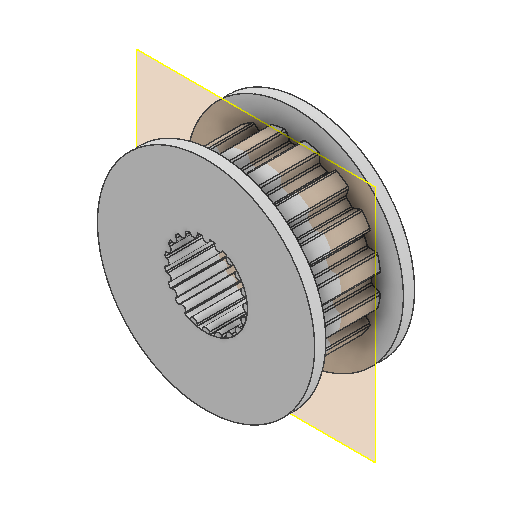
# Autodesk Inventor part: Diff Small Pulley
Saved by Autodesk Inventor 2025.2 (Build 292293000, 293)
## iProperties
Created: 2025-02-20
Part Number: Diff Small Pulley
Material: Generic
Document SubType Name: Modeling
Designer: Jakeg
Density: 1 g/cm^3
Appearance: Default
Author: Jakeg
Autodesk Inventor part; units mm, degrees
ref_plane "YZ Plane" through (0, 0, 0) normal (1, 0, 0) x (0, 1, 0)
ref_plane "XZ Plane" through (0, 0, 0) normal (0, 1, 0) x (-1, 0, 0)
ref_plane "XY Plane" through (0, 0, 0) normal (0, 0, 1) x (1, 0, 0)
sketch "Sketch1" plane through (0, 0, 0) normal (0, 0, 1) x (1, 0, 0)
  circle A0 centre (0, 0) radius 6
  circle A1 centre (0, 0) radius 15.75
  dimension "d0" = 12
  dimension "d1" = 31.5
  constraints: 2 centre point, 2 coincident
  measures "d0" diameter of A0
  measures "d1" diameter of A1
extrude "Extrusion1" add sketch "Sketch1" along normal blind 14.5
ref_plane "Work Plane1" through (0, 0, 7.25) normal (0, 0, 1) x (1, 0, 0)
sketch "Sketch2" plane through (0, 0, 7.25) normal (0, 0, 1) x (1, 0, 0)
  circle A0 centre (0, 0) radius 12.5
  circle A1 centre (0, 0) radius 15.75
  dimension "d5" = 25
  constraints: 2 centre point, 2 coincident
  measures "d5" diameter of A0
extrude "Extrusion2" cut sketch "Sketch2" along normal mid plane 11.25
sketch "Sketch3" plane through (0, 0, 14.5) normal (0, 0, 1) x (1, 0, 0)
  arc A0 (-1.277994, -5.546817) -> (-2.226914, -5.238494) centre (-1.827608, -5.623954) ccw
  arc A1 (-1.278569, -5.828822) -> (-1.277994, -5.546817) centre (-2.268289, -5.685804) ccw
  arc A2 (-1.278569, -5.828822) -> (-1.158554, -5.997554) centre (-1.130111, -5.850275) ccw
  arc A3 (-1.158554, -5.997554) -> (-0.751747, -6.061994) centre (0, 0) ccw
  arc A4 (-0.751747, -6.061994) -> (-0.585466, -5.938608) centre (-0.733287, -5.913134) ccw
  arc A5 (-0.498868, -5.670227) -> (-0.585466, -5.938608) centre (0.400009, -6.108429) ccw
  arc A6 (0.498885, -5.670227) -> (-0.498868, -5.670227) centre (0.000009, -5.913429) ccw
  arc A7 (0.585484, -5.938608) -> (0.498885, -5.670227) centre (-0.399991, -6.108429) ccw
  arc A8 (0.585484, -5.938608) -> (0.751765, -6.061994) centre (0.733305, -5.913134) ccw
  arc A9 (0.751765, -6.061994) -> (1.158327, -5.997601) centre (0.000009, 0.000071) ccw
  arc A10 (1.158327, -5.997601) -> (1.278342, -5.82887) centre (1.129884, -5.850323) ccw
  arc A11 (1.277768, -5.546864) -> (1.278342, -5.82887) centre (2.268062, -5.685851) ccw
  arc A12 (2.226687, -5.238541) -> (1.277768, -5.546864) centre (1.827381, -5.624002) ccw
  arc A13 (2.391981, -5.467026) -> (2.226687, -5.238541) centre (1.507217, -5.933065) ccw
  arc A14 (2.391981, -5.467026) -> (2.588253, -5.53299) centre (2.524696, -5.397121) ccw
  arc A15 (2.588253, -5.53299) -> (2.955018, -5.346114) centre (0.000009, 0.000071) ccw
  arc A16 (2.955018, -5.346114) -> (3.017017, -5.148554) centre (2.882455, -5.214833) ccw
  arc A17 (2.929327, -4.880528) -> (3.017017, -5.148554) centre (3.914102, -4.706695) ccw
  arc A18 (3.736526, -4.294064) -> (2.929327, -4.880528) centre (3.475877, -4.784051) ccw
  arc A19 (3.964336, -4.460287) -> (3.736526, -4.294064) centre (3.266888, -5.176923) ccw
  arc A20 (3.964336, -4.460287) -> (4.171385, -4.462372) centre (4.068953, -4.352792) ccw
  arc A21 (4.171385, -4.462372) -> (4.462451, -4.171305) centre (0.000009, 0.000071) ccw
  arc A22 (4.462451, -4.171305) -> (4.460367, -3.964256) centre (4.352872, -4.068873) ccw
  arc A23 (4.294144, -3.736446) -> (4.460367, -3.964256) centre (5.177003, -3.266808) ccw
  arc A24 (4.880608, -2.929247) -> (4.294144, -3.736446) centre (4.784131, -3.475797) ccw
  arc A25 (5.148634, -3.016938) -> (4.880608, -2.929247) centre (4.706775, -3.914022) ccw
  arc A26 (5.148634, -3.016938) -> (5.346194, -2.954938) centre (5.214913, -2.882375) ccw
  arc A27 (5.346194, -2.954938) -> (5.53307, -2.588173) centre (0.000009, 0.000071) ccw
  arc A28 (5.53307, -2.588173) -> (5.467106, -2.391901) centre (5.3972, -2.524616) ccw
  arc A29 (5.238621, -2.226607) -> (5.467106, -2.391901) centre (5.933144, -1.507137) ccw
  arc A30 (5.546944, -1.277688) -> (5.238621, -2.226607) centre (5.624082, -1.827301) ccw
  arc A31 (5.82895, -1.278262) -> (5.546944, -1.277688) centre (5.685931, -2.267982) ccw
  arc A32 (5.82895, -1.278262) -> (5.997681, -1.158248) centre (5.850402, -1.129804) ccw
  arc A33 (5.997681, -1.158248) -> (6.062074, -0.751685) centre (0.000009, 0.000071) ccw
  arc A34 (6.062074, -0.751685) -> (5.938687, -0.585404) centre (5.913214, -0.733225) ccw
  arc A35 (5.663912, -0.495883) -> (5.938687, -0.585404) centre (6.107819, 0.40019) ccw
  arc A36 (5.663912, 0.50187) -> (5.663912, -0.495883) centre (5.907114, 0.002993) ccw
  arc A37 (5.932293, 0.588468) -> (5.663912, 0.50187) centre (6.102114, -0.397007) ccw
  arc A38 (5.932293, 0.588468) -> (6.05568, 0.754749) centre (5.90682, 0.736289) ccw
  arc A39 (6.05568, 0.754749) -> (5.991286, 1.161312) centre (-0.006386, 0.002993) ccw
  arc A40 (5.991286, 1.161312) -> (5.822555, 1.281326) centre (5.844008, 1.132868) ccw
  arc A41 (5.540549, 1.280752) -> (5.822555, 1.281326) centre (5.679536, 2.271046) ccw
  arc A42 (5.232227, 2.229671) -> (5.540549, 1.280752) centre (5.617687, 1.830365) ccw
  arc A43 (5.460712, 2.394966) -> (5.232227, 2.229671) centre (5.92675, 1.510201) ccw
  arc A44 (5.460712, 2.394966) -> (5.526676, 2.591237) centre (5.390806, 2.52768) ccw
  arc A45 (5.526676, 2.591237) -> (5.339799, 2.958002) centre (-0.006386, 0.002993) ccw
  arc A46 (5.339799, 2.958002) -> (5.14224, 3.020002) centre (5.208519, 2.885439) ccw
  arc A47 (4.874214, 2.932311) -> (5.14224, 3.020002) centre (4.700381, 3.917086) ccw
  arc A48 (4.287749, 3.73951) -> (4.874214, 2.932311) centre (4.777736, 3.478861) ccw
  arc A49 (4.453973, 3.96732) -> (4.287749, 3.73951) centre (5.170609, 3.269873) ccw
  arc A50 (4.453973, 3.96732) -> (4.456057, 4.174369) centre (4.346477, 4.071937) ccw
  arc A51 (4.456057, 4.174369) -> (4.16499, 4.465436) centre (-0.006386, 0.002993) ccw
  arc A52 (4.16499, 4.465436) -> (3.957941, 4.463352) centre (4.062558, 4.355856) ccw
  arc A53 (3.730131, 4.297128) -> (3.957941, 4.463352) centre (3.260494, 5.179988) ccw
  arc A54 (2.922932, 4.883593) -> (3.730131, 4.297128) centre (3.469482, 4.787115) ccw
  arc A55 (3.010623, 5.151619) -> (2.922932, 4.883593) centre (3.907707, 4.709759) ccw
  arc A56 (3.010623, 5.151619) -> (2.948623, 5.349178) centre (2.87606, 5.217898) ccw
  arc A57 (2.948623, 5.349178) -> (2.581858, 5.536054) centre (-0.006386, 0.002993) ccw
  arc A58 (2.581858, 5.536054) -> (2.385587, 5.470091) centre (2.518301, 5.400185) ccw
  arc A59 (2.220292, 5.241606) -> (2.385587, 5.470091) centre (1.500822, 5.936129) ccw
  arc A60 (1.271373, 5.549928) -> (2.220292, 5.241606) centre (1.820986, 5.627066) ccw
  arc A61 (1.271947, 5.831934) -> (1.271373, 5.549928) centre (2.261667, 5.688915) ccw
  arc A62 (1.271947, 5.831934) -> (1.151933, 6.000665) centre (1.123489, 5.853387) ccw
  arc A63 (1.151933, 6.000665) -> (0.745371, 6.065058) centre (-0.006386, 0.002993) ccw
  arc A64 (0.745371, 6.065058) -> (0.579089, 5.941672) centre (0.72691, 5.916199) ccw
  arc A65 (0.492491, 5.673291) -> (0.579089, 5.941672) centre (-0.406386, 6.111493) ccw
  arc A66 (-0.505262, 5.673291) -> (0.492491, 5.673291) centre (-0.006386, 5.916493) ccw
  arc A67 (-0.591861, 5.941672) -> (-0.505262, 5.673291) centre (0.393614, 6.111493) ccw
  arc A68 (-0.591861, 5.941672) -> (-0.758142, 6.065058) centre (-0.739682, 5.916199) ccw
  arc A69 (-0.758142, 6.065058) -> (-1.164704, 6.000665) centre (-0.006386, 0.002993) ccw
  arc A70 (-1.164704, 6.000665) -> (-1.284719, 5.831934) centre (-1.136261, 5.853387) ccw
  arc A71 (-1.284144, 5.549928) -> (-1.284719, 5.831934) centre (-2.274439, 5.688915) ccw
  arc A72 (-2.233064, 5.241606) -> (-1.284144, 5.549928) centre (-1.833758, 5.627066) ccw
  arc A73 (-2.398358, 5.470091) -> (-2.233064, 5.241606) centre (-1.513593, 5.936129) ccw
  arc A74 (-2.398358, 5.470091) -> (-2.594629, 5.536054) centre (-2.531073, 5.400185) ccw
  arc A75 (-2.594629, 5.536054) -> (-2.961395, 5.349178) centre (-0.006386, 0.002993) ccw
  arc A76 (-2.961395, 5.349178) -> (-3.023394, 5.151619) centre (-2.888832, 5.217898) ccw
  arc A77 (-2.935704, 4.883593) -> (-3.023394, 5.151619) centre (-3.920479, 4.709759) ccw
  arc A78 (-3.742903, 4.297128) -> (-2.935704, 4.883593) centre (-3.482254, 4.787115) ccw
  arc A79 (-3.970713, 4.463352) -> (-3.742903, 4.297128) centre (-3.273265, 5.179988) ccw
  arc A80 (-3.970713, 4.463352) -> (-4.177762, 4.465436) centre (-4.07533, 4.355856) ccw
  arc A81 (-4.177762, 4.465436) -> (-4.468828, 4.174369) centre (-0.006386, 0.002993) ccw
  arc A82 (-4.468828, 4.174369) -> (-4.466744, 3.96732) centre (-4.359249, 4.071937) ccw
  arc A83 (-4.300521, 3.73951) -> (-4.466744, 3.96732) centre (-5.18338, 3.269873) ccw
  arc A84 (-4.886985, 2.932311) -> (-4.300521, 3.73951) centre (-4.790508, 3.478861) ccw
  arc A85 (-5.155011, 3.020002) -> (-4.886985, 2.932311) centre (-4.713152, 3.917086) ccw
  arc A86 (-5.155011, 3.020002) -> (-5.352571, 2.958002) centre (-5.22129, 2.885439) ccw
  arc A87 (-5.352571, 2.958002) -> (-5.539447, 2.591237) centre (-0.006386, 0.002993) ccw
  arc A88 (-5.539447, 2.591237) -> (-5.473483, 2.394966) centre (-5.403577, 2.52768) ccw
  arc A89 (-5.244998, 2.229671) -> (-5.473483, 2.394966) centre (-5.939521, 1.510201) ccw
  arc A90 (-5.553321, 1.280752) -> (-5.244998, 2.229671) centre (-5.630458, 1.830365) ccw
  arc A91 (-5.835326, 1.281326) -> (-5.553321, 1.280752) centre (-5.692308, 2.271046) ccw
  arc A92 (-5.835326, 1.281326) -> (-6.004058, 1.161312) centre (-5.856779, 1.132868) ccw
  arc A93 (-6.004058, 1.161312) -> (-6.068451, 0.754749) centre (-0.006386, 0.002993) ccw
  arc A94 (-6.068451, 0.754749) -> (-5.945064, 0.588468) centre (-5.919591, 0.736289) ccw
  arc A95 (-5.676683, 0.50187) -> (-5.945064, 0.588468) centre (-6.114886, -0.397007) ccw
  arc A96 (-5.676683, -0.495883) -> (-5.676683, 0.50187) centre (-5.919886, 0.002993) ccw
  arc A97 (-5.945064, -0.582482) -> (-5.676683, -0.495883) centre (-6.114886, 0.402993) ccw
  arc A98 (-5.945064, -0.582482) -> (-6.068451, -0.748763) centre (-5.919591, -0.730303) ccw
  arc A99 (-6.068451, -0.748763) -> (-6.004058, -1.155325) centre (-0.006386, 0.002993) ccw
  arc A100 (-6.004058, -1.155325) -> (-5.835326, -1.27534) centre (-5.856779, -1.126882) ccw
  arc A101 (-5.553321, -1.274765) -> (-5.835326, -1.27534) centre (-5.692308, -2.26506) ccw
  arc A102 (-5.244998, -2.223685) -> (-5.553321, -1.274765) centre (-5.630458, -1.824379) ccw
  arc A103 (-5.473483, -2.388979) -> (-5.244998, -2.223685) centre (-5.939521, -1.504214) ccw
  arc A104 (-5.473483, -2.388979) -> (-5.539447, -2.585251) centre (-5.403577, -2.521694) ccw
  arc A105 (-5.539447, -2.585251) -> (-5.352571, -2.952016) centre (-0.006386, 0.002993) ccw
  arc A106 (-5.352571, -2.952016) -> (-5.155011, -3.014015) centre (-5.22129, -2.879453) ccw
  arc A107 (-4.886985, -2.926325) -> (-5.155011, -3.014015) centre (-4.713152, -3.9111) ccw
  arc A108 (-4.300521, -3.733524) -> (-4.886985, -2.926325) centre (-4.790508, -3.472875) ccw
  arc A109 (-4.466744, -3.961334) -> (-4.300521, -3.733524) centre (-5.18338, -3.263886) ccw
  arc A110 (-4.466744, -3.961334) -> (-4.468828, -4.168383) centre (-4.359249, -4.065951) ccw
  arc A111 (-4.468828, -4.168383) -> (-4.177762, -4.459449) centre (-0.006386, 0.002993) ccw
  arc A112 (-4.177762, -4.459449) -> (-3.970713, -4.457365) centre (-4.07533, -4.34987) ccw
  arc A113 (-3.742903, -4.291142) -> (-3.970713, -4.457365) centre (-3.273265, -5.174001) ccw
  arc A114 (-2.935704, -4.877606) -> (-3.742903, -4.291142) centre (-3.482254, -4.781129) ccw
  arc A115 (-3.023394, -5.145632) -> (-2.935704, -4.877606) centre (-3.920479, -4.703773) ccw
  arc A116 (-3.023394, -5.145632) -> (-2.961395, -5.343192) centre (-2.888832, -5.211911) ccw
  arc A117 (-2.961395, -5.343192) -> (-2.58848, -5.532943) centre (-0.005971, 0.003744) ccw
  arc A118 (-2.58848, -5.532943) -> (-2.392208, -5.466979) centre (-2.524923, -5.397073) ccw
  arc A119 (-2.226914, -5.238494) -> (-2.392208, -5.466979) centre (-1.507443, -5.933017) ccw
  circle A120 centre (-0.005971, 0.003744) radius 6
  circle A121 centre (-0.005971, 0.003744) radius 12.520387
  arc A122 (-9.716442, 7.90734) -> (-9.702841, 7.703356) centre (-9.600106, 7.812651) ccw
  arc A123 (-9.536618, 7.475546) -> (-9.702841, 7.703356) centre (-10.419477, 7.005908) ccw
  arc A124 (-10.123082, 6.668347) -> (-9.536618, 7.475546) centre (-10.026605, 7.214897) ccw
  arc A125 (-10.391108, 6.756038) -> (-10.123082, 6.668347) centre (-9.949249, 7.653122) ccw
  arc A126 (-10.391108, 6.756038) -> (-10.584118, 6.70172) centre (-10.457387, 6.621475) ccw
  arc A127 (-11.383003, 4.903875) -> (-11.564057, 4.817719) centre (-11.425588, 4.760046) ccw
  arc A128 (-11.383003, 4.903875) -> (-11.104013, 4.862742) centre (-11.099108, 5.86273) ccw
  arc A129 (-11.104013, 4.862742) -> (-10.662401, 5.757443) centre (-11.10129, 5.417735) ccw
  arc A130 (-10.912613, 6.152636) -> (-10.864734, 5.953884) centre (-10.781948, 6.07897) ccw
  arc A131 (-10.662401, 5.757443) -> (-10.864734, 5.953884) centre (-11.453193, 5.145357) ccw
  arc A132 (-12.047614, 2.910722) -> (-12.211503, 2.795208) centre (-12.065279, 2.761766) ccw
  arc A133 (-12.047614, 2.910722) -> (-11.765685, 2.917331) centre (-11.929849, 3.903764) ccw
  arc A134 (-11.765685, 2.917331) -> (-11.481631, 3.873795) centre (-11.856796, 3.464801) ccw
  arc A135 (-11.795031, 4.221017) -> (-11.714252, 4.033216) centre (-11.653796, 4.170494) ccw
  arc A136 (-11.481631, 3.873795) -> (-11.714252, 4.033216) centre (-12.157604, 3.136869) ccw
  arc A137 (-12.36582, 0.83392) -> (-12.50783, 0.692369) centre (-12.358057, 0.684121) ccw
  arc A138 (-12.36582, 0.83392) -> (-12.089064, 0.888079) centre (-12.417575, 1.83258) ccw
  arc A139 (-12.089064, 0.888079) -> (-11.970739, 1.878791) centre (-12.271387, 1.412277) ccw
  arc A140 (-12.338312, 2.168054) -> (-12.226956, 1.996606) centre (-12.19057, 2.142126) ccw
  arc A141 (-11.970739, 1.878791) -> (-12.226956, 1.996606) centre (-12.512448, 1.038225) ccw
  arc A142 (-12.328468, -1.266787) -> (-12.444514, -1.430301) centre (-12.295501, -1.413119) ccw
  arc A143 (-12.328468, -1.266787) -> (-12.064846, -1.166634) centre (-12.548252, -0.291239) ccw
  arc A144 (-12.064846, -1.166634) -> (-12.115654, -0.170176) centre (-12.333136, -0.68079) ccw
  arc A145 (-12.526825, 0.052806) -> (-12.388096, -0.097357) centre (-12.376826, 0.05222) ccw
  arc A146 (-12.115654, -0.170176) -> (-12.388096, -0.097357) centre (-12.507514, -1.090201) ccw
  arc A147 (-11.936633, -3.330965) -> (-12.023374, -3.511738) centre (-11.879409, -3.46962) ccw
  arc A148 (-11.936633, -3.330965) -> (-11.693728, -3.1877) centre (-12.318124, -2.406592) ccw
  arc A149 (-11.693728, -3.1877) -> (-11.912207, -2.214161) centre (-12.040267, -2.754185) ccw
  arc A150 (-12.355149, -2.063875) -> (-12.193038, -2.188432) centre (-12.207208, -2.039103) ccw
  arc A151 (-11.912207, -2.214161) -> (-12.193038, -2.188432) centre (-12.142946, -3.187177) ccw
  arc A152 (-11.201585, -5.29923) -> (-11.256529, -5.492063) centre (-11.121752, -5.426221) ccw
  arc A153 (-11.201585, -5.29923) -> (-10.986386, -5.116975) centre (-11.733809, -4.452626) ccw
  arc A154 (-10.986386, -5.116975) -> (-11.366252, -4.194363) centre (-11.401206, -4.748261) ccw
  arc A155 (-11.82822, -4.121096) -> (-11.647391, -4.216465) centre (-11.686594, -4.071678) ccw
  arc A156 (-11.366252, -4.194363) -> (-11.647391, -4.216465) centre (-11.429232, -5.192378) ccw
  arc A157 (-10.144472, -7.11496) -> (-10.166036, -7.314305) centre (-10.044326, -7.226632) ccw
  arc A158 (-10.144472, -7.11496) -> (-9.96317, -6.898958) centre (-10.812117, -6.37048) ccw
  arc A159 (-9.96317, -6.898958) -> (-10.493494, -6.053815) centre (-10.434336, -6.605653) ccw
  arc A160 (-10.9612, -6.059674) -> (-10.766854, -6.123111) centre (-10.829962, -5.987033) ccw
  arc A161 (-10.493494, -6.053815) -> (-10.766854, -6.123111) centre (-10.386902, -7.048118) ccw
  arc A162 (-8.795705, -8.72592) -> (-8.78327, -8.926042) centre (-8.678126, -8.819061) ccw
  arc A163 (-8.795705, -8.72592) -> (-8.653515, -8.482384) centre (-9.579564, -8.104981) ccw
  arc A164 (-8.653515, -8.482384) -> (-9.319041, -7.739023) centre (-9.167472, -8.272926) ccw
  arc A165 (-9.779029, -7.823841) -> (-9.576758, -7.853521) centre (-9.661956, -7.730065) ccw
  arc A166 (-9.319041, -7.739023) -> (-9.576758, -7.853521) centre (-9.045944, -8.70101) ccw
  arc A167 (-7.194085, -10.085765) -> (-7.148008, -10.280906) centre (-7.062457, -10.157695) ccw
  arc A168 (-7.194085, -10.085765) -> (-7.095098, -9.821702) centre (-8.071608, -9.60623) ccw
  arc A169 (-7.095098, -9.821702) -> (-7.87668, -9.201508) centre (-7.637061, -9.702115) ccw
  arc A170 (-8.315717, -9.362844) -> (-8.111339, -9.357913) centre (-8.216176, -9.250631) ccw
  arc A171 (-7.87668, -9.201508) -> (-8.111339, -9.357913) centre (-7.444935, -10.103503) ccw
  arc A172 (-5.385688, -11.155374) -> (-5.307295, -11.339922) centre (-5.243797, -11.204025) ccw
  arc A173 (-5.385688, -11.155374) -> (-5.332752, -10.878381) centre (-6.331631, -10.83104) ccw
  arc A174 (-5.332752, -10.878381) -> (-6.207905, -10.399195) centre (-5.88713, -10.852107) ccw
  arc A175 (-6.61336, -10.632409) -> (-6.412756, -10.593008) centre (-6.534215, -10.504988) ccw
  arc A176 (-6.207905, -10.399195) -> (-6.412756, -10.593008) centre (-5.629932, -11.215252) ccw
  arc A177 (-3.422539, -11.903978) -> (-3.314084, -12.072622) centre (-3.274466, -11.927949) ccw
  arc A178 (-3.422539, -11.903978) -> (-3.417176, -11.622023) centre (-4.409688, -11.744174) ccw
  arc A179 (-3.417176, -11.622023) -> (-4.360723, -11.297631) centre (-3.96802, -11.689816) ccw
  arc A180 (-4.720933, -11.596012) -> (-4.529873, -11.523276) centre (-4.664461, -11.457049) ccw
  arc A181 (-4.360723, -11.297631) -> (-4.529873, -11.523276) centre (-3.65315, -12.004271) ccw
  arc A182 (-1.361113, -12.31004) -> (-1.225717, -12.457929) centre (-1.211119, -12.308641) ccw
  arc A183 (-1.361113, -12.31004) -> (-1.403478, -12.031234) centre (-2.361069, -12.319363) ccw
  arc A184 (-1.403478, -12.031234) -> (-2.388275, -11.870968) centre (-1.934941, -12.191145) ccw
  arc A185 (-2.692878, -12.225933) -> (-2.516858, -12.121955) centre (-2.660702, -12.079425) ccw
  arc A186 (-2.388275, -11.870968) -> (-2.516858, -12.121955) centre (-1.571457, -12.447864) ccw
  arc A187 (0.739287, -12.361878) -> (0.897728, -12.484758) centre (0.886886, -12.335151) ccw
  arc A188 (0.739287, -12.361878) -> (0.650412, -12.094242) centre (-0.244711, -12.54006) ccw
  arc A189 (0.650412, -12.094242) -> (-0.347304, -12.102714) centre (0.153619, -12.341671) ccw
  arc A190 (-0.587536, -12.504051) -> (-0.431621, -12.37182) centre (-0.580584, -12.354212) ccw
  arc A191 (-0.347304, -12.102714) -> (-0.431621, -12.37182) centre (0.55526, -12.533268) ccw
  arc A192 (2.818234, -12.058001) -> (2.995163, -12.152337) centre (2.959194, -12.006714) ccw
  arc A193 (2.818234, -12.058001) -> (2.685408, -11.809235) centre (1.878504, -12.399917) ccw
  arc A194 (2.685408, -11.809235) -> (1.703474, -11.9862) centre (2.237576, -12.137064) ccw
  arc A195 (1.534524, -12.422363) -> (1.665849, -12.265685) centre (1.516053, -12.273505) ccw
  arc A196 (1.703474, -11.9862) -> (1.665849, -12.265685) centre (2.66582, -12.258027) ccw
  arc A197 (4.815922, -11.407152) -> (5.00625, -11.47023) centre (4.946187, -11.33278) ccw
  arc A198 (4.815922, -11.407152) -> (4.642965, -11.184411) centre (3.947493, -11.902965) ccw
  arc A199 (4.642965, -11.184411) -> (3.705062, -11.524778) centre (4.256978, -11.583209) ccw
  arc A200 (3.612255, -11.983221) -> (3.715212, -11.806602) centre (3.568893, -11.839625) ccw
  arc A201 (3.705062, -11.524778) -> (3.715212, -11.806602) centre (4.699505, -11.630058) ccw
  arc A202 (6.674882, -10.428053) -> (6.873132, -10.458058) centre (6.790704, -10.332736) ccw
  arc A203 (6.674882, -10.428053) -> (6.466769, -10.237747) centre (5.902737, -11.0635) ccw
  arc A204 (6.466769, -10.237747) -> (5.599879, -10.731724) centre (6.153731, -10.69604) ccw
  arc A205 (5.585884, -11.199257) -> (5.657512, -11.007779) centre (5.518878, -11.065055) ccw
  arc A206 (5.599879, -10.731724) -> (5.657512, -11.007779) centre (6.59781, -10.667428) ccw
  arc A207 (8.341633, -9.148872) -> (8.542102, -9.144942) centre (8.43968, -9.035353) ccw
  arc A208 (8.341633, -9.148872) -> (8.104352, -8.996475) centre (7.687986, -9.905672) ccw
  arc A209 (8.104352, -8.996475) -> (7.333414, -9.629851) centre (7.873269, -9.501079) ccw
  arc A210 (7.398634, -10.093025) -> (7.436871, -9.892195) centre (7.309911, -9.972077) ccw
  arc A211 (7.333414, -9.629851) -> (7.436871, -9.892195) centre (8.306125, -9.397829) ccw
  arc A212 (9.768227, -7.606409) -> (9.965149, -7.568655) centre (9.845679, -7.477952) ccw
  arc A213 (9.768227, -7.606409) -> (9.508604, -7.496304) centre (9.251882, -8.462789) ccw
  arc A214 (9.508604, -7.496304) -> (8.855797, -8.25086) centre (9.366123, -8.032703) ccw
  arc A215 (8.998355, -8.696348) -> (9.002102, -8.491946) centre (8.890468, -8.592135) ccw
  arc A216 (8.855797, -8.25086) -> (9.002102, -8.491946) centre (9.775304, -7.857786) ccw
  arc A217 (10.913624, -5.845037) -> (11.101332, -5.774547) centre (10.968252, -5.705338) ccw
  arc A218 (10.913624, -5.845037) -> (10.639127, -5.780393) centre (10.549434, -6.776362) ccw
  arc A219 (10.639127, -5.780393) -> (10.12323, -6.634419) centre (10.589347, -6.333156) ccw
  arc A220 (10.339025, -7.049408) -> (10.308175, -6.847312) centre (10.215078, -6.964926) ccw
  arc A221 (10.12323, -6.634419) -> (10.308175, -6.847312) centre (10.963081, -6.091602) ccw
  arc A222 (11.744871, -3.915428) -> (11.917967, -3.814229) centre (11.775105, -3.768506) ccw
  arc A223 (11.744871, -3.915428) -> (11.463398, -3.898104) centre (11.543315, -4.894905) ccw
  arc A224 (11.463398, -3.898104) -> (11.099253, -4.827033) centre (11.507752, -4.451328) ccw
  arc A225 (11.382078, -5.199582) -> (11.317516, -5.005607) centre (11.245636, -5.137263) ccw
  arc A226 (11.099253, -4.827033) -> (11.317516, -5.005607) centre (11.835287, -4.150088) ccw
  arc A227 (12.238057, -1.873093) -> (12.391559, -1.744096) centre (12.243025, -1.723175) ccw
  arc A228 (12.238057, -1.873093) -> (11.957704, -1.903587) centre (12.204932, -2.872544) ccw
  arc A229 (11.957704, -1.903587) -> (11.755787, -2.880695) centre (12.094915, -2.441358) ccw
  arc A230 (12.097504, -3.200088) -> (12.00109, -3.019814) centre (11.952493, -3.161724) ccw
  arc A231 (11.755787, -2.880695) -> (12.00109, -3.019814) centre (12.366829, -2.089097) ccw
  arc A232 (12.378992, 0.223214) -> (12.508486, 0.376297) centre (12.358553, 0.371815) ccw
  arc A233 (12.378992, 0.223214) -> (12.107825, 0.145778) centre (12.515252, -0.76746) ccw
  arc A234 (12.107825, 0.145778) -> (12.073945, -0.851399) centre (12.333947, -0.361069) ccw
  arc A235 (12.464724, -1.108448) -> (12.33923, -0.947061) centre (12.315316, -1.095142) ccw
  arc A236 (12.073945, -0.851399) -> (12.33923, -0.947061) centre (12.542417, 0.032079) ccw
  arc A237 (12.163622, 2.313185) -> (12.265382, 2.485951) centre (12.118363, 2.456194) ccw
  arc A238 (12.163622, 2.313185) -> (11.909442, 2.191036) centre (12.465346, 1.35979) ccw
  arc A239 (11.909442, 2.191036) -> (12.044573, 1.202476) centre (12.217969, 1.729694) ccw
  arc A240 (12.473173, 1.015167) -> (12.32221, 1.153024) centre (12.323665, 1.003031) ccw
  arc A241 (12.044573, 1.202476) -> (12.32221, 1.153024) centre (12.356998, 2.152419) ccw
  arc A242 (11.598143, 4.336696) -> (11.669242, 4.524175) centre (11.529367, 4.469999) ccw
  arc A243 (11.598143, 4.336696) -> (11.368263, 4.173348) centre (12.056652, 3.448006) ccw
  arc A244 (11.368263, 4.173348) -> (11.668517, 3.221845) centre (11.750319, 3.770783) ccw
  arc A245 (12.122608, 3.109664) -> (11.950518, 3.220025) centre (11.977301, 3.072435) ccw
  arc A246 (11.668517, 3.221845) -> (11.950518, 3.220025) centre (11.815908, 4.210923) ccw
  arc A247 (10.698823, 6.235535) -> (10.737215, 6.432332) centre (10.608508, 6.355297) ccw
  arc A248 (10.698823, 6.235535) -> (10.499856, 6.035686) centre (11.300926, 5.437116) ccw
  arc A249 (10.499856, 6.035686) -> (10.956596, 5.148613) centre (10.94445, 5.70348) ccw
  arc A250 (11.423114, 5.114787) -> (11.234848, 5.194477) centre (11.286189, 5.053537) ccw
  arc A251 (10.956596, 5.148613) -> (11.234848, 5.194477) centre (10.934711, 6.148373) ccw
  arc A252 (9.491534, 7.955074) -> (9.496115, 8.155529) centre (9.382278, 8.057851) ccw
  arc A253 (9.491534, 7.955074) -> (9.329203, 7.724474) centre (10.21991, 7.269896) ccw
  arc A254 (9.329203, 7.724474) -> (9.92929, 6.92735) centre (9.823545, 7.472184) ccw
  arc A255 (10.394813, 6.972853) -> (10.195788, 7.01958) centre (10.270209, 6.889344) ccw
  arc A256 (9.92929, 6.92735) -> (10.195788, 7.01958) centre (9.738759, 7.909032) ccw
  arc A257 (8.011007, 9.445847) -> (7.981645, 9.644193) centre (7.885953, 9.528681) ccw
  arc A258 (8.011007, 9.445847) -> (7.889982, 9.19113) centre (8.844701, 8.893621) ccw
  arc A259 (7.889982, 9.19113) -> (8.616152, 8.506887) centre (8.419851, 9.026012) ccw
  arc A260 (9.06729, 8.630409) -> (8.86323, 8.642828) centre (8.958591, 8.527043) ccw
  arc A261 (8.616152, 8.506887) -> (8.86323, 8.642828) centre (8.262457, 9.442248) ccw
  arc A262 (6.299834, 10.664966) -> (6.237373, 10.855497) centre (6.162579, 10.725474) ccw
  arc A263 (6.299834, 10.664966) -> (6.223598, 10.39346) centre (7.214863, 10.261578) ccw
  arc A264 (6.223598, 10.39346) -> (7.054959, 9.841782) centre (6.77375, 10.320265) ccw
  arc A265 (7.478733, 10.03977) -> (7.275509, 10.017524) centre (7.389067, 9.919521) ccw
  arc A266 (7.054959, 9.841782) -> (7.275509, 10.017524) centre (6.548276, 10.703914) ccw
  arc A267 (4.407243, 11.577359) -> (4.313481, 11.754594) centre (4.261736, 11.613801) ccw
  arc A268 (4.407243, 11.577359) -> (4.377988, 11.296875) centre (5.377283, 11.334415) ccw
  arc A269 (4.377988, 11.296875) -> (5.290625, 10.893633) centre (4.932596, 11.317709) ccw
  arc A270 (5.674842, 11.160392) -> (5.478302, 11.104121) centre (5.606789, 11.026718) ccw
  arc A271 (5.290625, 10.893633) -> (5.478302, 11.104121) centre (4.645528, 11.657734) ccw
  arc A272 (2.387679, 12.15678) -> (2.265313, 12.315619) centre (2.238107, 12.168106) ccw
  arc A273 (2.387679, 12.15678) -> (2.406247, 11.875385) centre (3.384824, 12.081267) ccw
  arc A274 (2.406247, 11.875385) -> (3.373905, 11.632181) centre (2.949357, 11.989649) ccw
  arc A275 (3.707514, 11.960035) -> (3.52331, 11.871358) centre (3.66303, 11.816783) ccw
  arc A276 (3.373905, 11.632181) -> (3.52331, 11.871358) centre (2.608954, 12.276269) ccw
  arc A277 (0.299243, 12.386557) -> (0.151793, 12.522432) centre (0.149908, 12.372443) ccw
  arc A278 (0.299243, 12.386557) -> (0.3651, 12.112348) centre (1.294806, 12.480649) ccw
  arc A279 (0.3651, 12.112348) -> (1.359941, 12.036177) centre (0.881087, 12.316755) ccw
  arc A280 (1.633343, 12.415696) -> (1.466775, 12.297164) centre (1.613708, 12.266986) ccw
  arc A281 (1.359941, 12.036177) -> (1.466775, 12.297164) centre (0.497141, 12.541723) ccw
  arc A282 (-1.797986, 12.260082) -> (-1.966278, 12.369083) centre (-1.942787, 12.220934) ccw
  arc A283 (-1.797986, 12.260082) -> (-1.686735, 12.000948) centre (-0.832644, 12.521072) ccw
  arc A284 (-1.686735, 12.000948) -> (-0.693331, 12.094001) centre (-1.212715, 12.289617) ccw
  arc A285 (-0.488, 12.514266) -> (-0.63214, 12.369289) centre (-0.48222, 12.364377) ccw
  arc A286 (-0.693331, 12.094001) -> (-0.63214, 12.369289) centre (-1.629157, 12.446462) ccw
  arc A287 (-3.843673, 11.780993) -> (-4.027966, 11.859985) centre (-3.979776, 11.717937) ccw
  arc A288 (-3.843673, 11.780993) -> (-3.690229, 11.544388) centre (-2.936325, 12.201372) ccw
  arc A289 (-3.690229, 11.544388) -> (-2.72684, 11.803989) centre (-3.271812, 11.909014) ccw
  arc A290 (-2.595488, 12.252909) -> (-2.713053, 12.085658) centre (-2.56446, 12.106153) ccw
  arc A291 (-2.72684, 11.803989) -> (-2.713053, 12.085658) centre (-3.708772, 11.993224) ccw
  arc A292 (-5.778969, 10.963073) -> (-5.97396, 11.009783) centre (-5.902457, 10.877922) ccw
  arc A293 (-5.778969, 10.963073) -> (-5.587745, 10.755803) centre (-4.955716, 11.530748) ccw
  arc A294 (-5.587745, 10.755803) -> (-4.682087, 11.174483) centre (-5.236969, 11.185897) ccw
  arc A295 (-4.628492, 11.639145) -> (-4.7161, 11.454431) centre (-4.573108, 11.499744) ccw
  arc A296 (-4.682087, 11.174483) -> (-4.7161, 11.454431) centre (-5.681875, 11.195049) ccw
  arc A297 (-7.548198, 9.829851) -> (-7.748279, 9.842935) centre (-7.655519, 9.725055) ccw
  arc A298 (-7.548198, 9.829851) -> (-7.324696, 9.657879) centre (-6.832725, 10.52849) ccw
  arc A299 (-7.324696, 9.657879) -> (-6.502822, 10.223594) centre (-7.051652, 10.141068) ccw
  arc A300 (-6.528526, 10.69063) -> (-6.583658, 10.493767) centre (-6.45038, 10.562594) ccw
  arc A301 (-6.502822, 10.223594) -> (-6.583658, 10.493767) centre (-7.491705, 10.074899) ccw
  arc A302 (-9.100463, 8.413928) -> (-9.299877, 8.39301) centre (-9.18853, 8.292502) ccw
  arc A303 (-9.100463, 8.413928) -> (-8.851112, 8.282202) centre (-8.513352, 9.223434) ccw
  arc A304 (-8.851112, 8.282202) -> (-8.136666, 8.978677) centre (-8.663655, 8.804586) ccw
  arc A305 (-8.24093, 9.434651) -> (-8.261999, 9.231302) centre (-8.14227, 9.321663) ccw
  arc A306 (-8.136666, 8.978677) -> (-8.261999, 9.231302) centre (-9.086196, 8.664999) ccw
  point P0 (-3.996075, -4.477223)
  point P1 (-3.034437, -5.175869)
  point P2 (-5.18537, -3.025088)
  point P3 (-4.486617, -3.986721)
  point P4 (-5.867799, -1.276476)
  point P5 (-5.50033, -2.407069)
  point P6 (-5.976518, 0.597512)
  point P7 (-5.976375, -0.591466)
  point P8 (-5.50081, 2.413462)
  point P9 (-5.868133, 1.282438)
  point P10 (-4.487164, 3.993594)
  point P11 (-5.186138, 3.031262)
  point P12 (-3.034756, 5.18317)
  point P13 (-3.997071, 4.483824)
  point P14 (-1.285757, 5.865667)
  point P15 (-2.417261, 5.497893)
  point P16 (0.588584, 5.974213)
  point P17 (-0.601322, 5.974134)
  point P18 (2.404717, 5.498158)
  point P19 (1.27297, 5.865852)
  point P20 (3.984793, 4.484124)
  point P21 (3.022086, 5.183597)
  point P22 (5.174095, 3.031436)
  point P23 (4.47473, 3.994147)
  point P24 (5.856206, 1.282371)
  point P25 (5.488642, 2.413978)
  point P26 (5.964359, -0.592214)
  point P27 (5.964544, 0.597841)
  point P28 (5.488898, -2.405908)
  point P29 (5.855147, -1.279729)
  point P30 (4.476789, -3.984347)
  point P31 (5.17271, -3.026316)
  point P32 (3.026633, -5.173448)
  point P33 (3.984588, -4.476819)
  point P34 (1.27974, -5.856883)
  point P35 (2.406739, -5.489782)
  point P36 (-0.593457, -5.967425)
  point P37 (0.593035, -5.96628)
  point P38 (-2.41007, -5.493556)
  point P39 (-1.279829, -5.859471)
  dimension "d8" = 0
  dimension "d9" = 0
  dimension "d20" = 360
  constraints: 612 point on circle, 306 centre point, 3 coincident, 2 tangent, 595 other
  measures "d8" distance of point (0, 0) point (0, 0)
  measures "d9" distance of point (0, 0) point (0, 0)
extrude "Extrusion3" add sketch "Sketch3" against normal blind 14.5 contours A1 A2 A120 A118 A119 A0 | A120 A4 A3 A2 | A118 A117 A116 A120 | A4 A5 A6 A7 A8 A120 | A120 A112 A113 A114 A115 A116 | A120 A10 A9 A8 | A112 A111 A110 A120 | A10 A11 A12 A13 A14 A120 | A120 A106 A107 A108 A109 A110 | A120 A16 A15 A14 | A106 A105 A104 A120 | A16 A17 A18 A19 A20 A120 | A120 A100 A101 A102 A103 A104 | A120 A22 A21 A20 | A100 A99 A98 A120 | A22 A23 A24 A25 A26 A120 | A120 A94 A95 A96 A97 A98 | A120 A28 A27 A26 | A94 A93 A92 A120 | A28 A29 A30 A31 A32 A120 | A120 A88 A89 A90 A91 A92 | A120 A34 A33 A32 | A88 A87 A86 A120 | A34 A35 A36 A37 A38 A120 | A120 A82 A83 A84 A85 A86 | A82 A81 A80 A120 | A120 A40 A39 A38 | A120 A76 A77 A78 A79 A80 | A40 A41 A42 A43 A44 A120 | A76 A75 A74 A120 | A120 A46 A45 A44 | A120 A70 A71 A72 A73 A74 | A46 A47 A48 A49 A50 A120 | A70 A69 A68 A120 | A120 A52 A51 A50 | A120 A64 A65 A66 A67 A68 | A52 A53 A54 A55 A56 A120 | A64 A63 A62 A120 | A120 A58 A57 A56 | A120 A58 A59 A60 A61 A62
sketch "Sketch6" plane through (0, 0, 1.625) normal (0, 0, 1) x (1, 0, 0)
  circle A0 centre (0, 0) radius 14.749764
  line L0 (3.580906, 11.795698) -> (3.627023, 10.739445)
  arc A1 (3.627023, 10.739445) -> (3.783579, 10.515859) centre (3.880781, 10.750524) ccw
  line L1 (3.783579, 10.515859) -> (4.760441, 10.11123)
  arc A2 (4.760441, 10.11123) -> (5.029242, 10.158627) centre (4.857642, 10.345895) ccw
  line L2 (5.029242, 10.158627) -> (5.808735, 10.872901)
  arc A3 (6.104383, 10.907281) -> (5.808735, 10.872901) centre (5.980335, 10.685632) ccw
  arc A4 (7.740967, 9.81375) -> (6.104383, 10.907281) centre (0, 0) ccw
  arc A5 (7.822344, 9.527451) -> (7.740967, 9.81375) centre (7.583662, 9.614324) ccw
  line L3 (7.822344, 9.527451) -> (7.46074, 8.533952)
  arc A6 (7.46074, 8.533952) -> (7.519817, 8.267474) centre (7.699422, 8.447079) ccw
  line L4 (7.519817, 8.267474) -> (8.267474, 7.519817)
  arc A7 (8.267474, 7.519817) -> (8.533952, 7.46074) centre (8.447079, 7.699422) ccw
  line L5 (8.533952, 7.46074) -> (9.527451, 7.822344)
  arc A8 (9.81375, 7.740967) -> (9.527451, 7.822344) centre (9.614324, 7.583662) ccw
  arc A9 (10.907281, 6.104383) -> (9.81375, 7.740967) centre (0, 0) ccw
  arc A10 (10.872901, 5.808735) -> (10.907281, 6.104383) centre (10.685632, 5.980335) ccw
  line L6 (10.872901, 5.808735) -> (10.158627, 5.029242)
  arc A11 (10.158627, 5.029242) -> (10.11123, 4.760441) centre (10.345895, 4.857642) ccw
  line L7 (10.11123, 4.760441) -> (10.515859, 3.783579)
  arc A12 (10.515859, 3.783579) -> (10.739445, 3.627023) centre (10.750524, 3.880781) ccw
  line L8 (10.739445, 3.627023) -> (11.795698, 3.580906)
  arc A13 (12.029063, 3.396161) -> (11.795698, 3.580906) centre (11.784619, 3.327148) ccw
  arc A14 (12.41306, 1.465679) -> (12.029063, 3.396161) centre (0, 0) ccw
  arc A15 (12.268157, 1.205693) -> (12.41306, 1.465679) centre (12.160812, 1.435895) ccw
  line L9 (12.268157, 1.205693) -> (11.309955, 0.758876)
  arc A16 (11.309955, 0.758876) -> (11.1633, 0.528673) centre (11.4173, 0.528673) ccw
  line L10 (11.1633, 0.528673) -> (11.1633, -0.528673)
  arc A17 (11.1633, -0.528673) -> (11.309955, -0.758876) centre (11.4173, -0.528673) ccw
  line L11 (11.309955, -0.758876) -> (12.268157, -1.205693)
  arc A18 (12.41306, -1.465679) -> (12.268157, -1.205693) centre (12.160812, -1.435895) ccw
  arc A19 (12.029063, -3.396161) -> (12.41306, -1.465679) centre (0, 0) ccw
  arc A20 (11.795698, -3.580906) -> (12.029063, -3.396161) centre (11.784619, -3.327148) ccw
  line L12 (11.795698, -3.580906) -> (10.739445, -3.627023)
  arc A21 (10.739445, -3.627023) -> (10.515859, -3.783579) centre (10.750524, -3.880781) ccw
  line L13 (10.515859, -3.783579) -> (10.11123, -4.760441)
  arc A22 (10.11123, -4.760441) -> (10.158627, -5.029242) centre (10.345895, -4.857642) ccw
  line L14 (10.158627, -5.029242) -> (10.872901, -5.808735)
  arc A23 (10.907281, -6.104383) -> (10.872901, -5.808735) centre (10.685632, -5.980335) ccw
  arc A24 (9.81375, -7.740967) -> (10.907281, -6.104383) centre (0, 0) ccw
  arc A25 (9.527451, -7.822344) -> (9.81375, -7.740967) centre (9.614324, -7.583662) ccw
  line L15 (9.527451, -7.822344) -> (8.533952, -7.46074)
  arc A26 (8.533952, -7.46074) -> (8.267474, -7.519817) centre (8.447079, -7.699422) ccw
  line L16 (8.267474, -7.519817) -> (7.519817, -8.267474)
  arc A27 (7.519817, -8.267474) -> (7.46074, -8.533952) centre (7.699422, -8.447079) ccw
  line L17 (7.46074, -8.533952) -> (7.822344, -9.527451)
  arc A28 (7.740967, -9.81375) -> (7.822344, -9.527451) centre (7.583662, -9.614324) ccw
  arc A29 (6.104383, -10.907281) -> (7.740967, -9.81375) centre (0, 0) ccw
  arc A30 (5.808735, -10.872901) -> (6.104383, -10.907281) centre (5.980335, -10.685632) ccw
  line L18 (5.808735, -10.872901) -> (5.029242, -10.158627)
  arc A31 (5.029242, -10.158627) -> (4.760441, -10.11123) centre (4.857642, -10.345895) ccw
  line L19 (4.760441, -10.11123) -> (3.783579, -10.515859)
  arc A32 (3.783579, -10.515859) -> (3.627023, -10.739445) centre (3.880781, -10.750524) ccw
  line L20 (3.627023, -10.739445) -> (3.580906, -11.795698)
  arc A33 (3.396161, -12.029063) -> (3.580906, -11.795698) centre (3.327148, -11.784619) ccw
  arc A34 (1.465679, -12.41306) -> (3.396161, -12.029063) centre (0, 0) ccw
  arc A35 (1.205693, -12.268157) -> (1.465679, -12.41306) centre (1.435895, -12.160812) ccw
  line L21 (1.205693, -12.268157) -> (0.758876, -11.309955)
  arc A36 (0.758876, -11.309955) -> (0.528673, -11.1633) centre (0.528673, -11.4173) ccw
  line L22 (0.528673, -11.1633) -> (-0.528673, -11.1633)
  arc A37 (-0.528673, -11.1633) -> (-0.758876, -11.309955) centre (-0.528673, -11.4173) ccw
  line L23 (-0.758876, -11.309955) -> (-1.205693, -12.268157)
  arc A38 (-1.465679, -12.41306) -> (-1.205693, -12.268157) centre (-1.435895, -12.160812) ccw
  arc A39 (-3.396161, -12.029063) -> (-1.465679, -12.41306) centre (0, 0) ccw
  arc A40 (-3.580906, -11.795698) -> (-3.396161, -12.029063) centre (-3.327148, -11.784619) ccw
  line L24 (-3.580906, -11.795698) -> (-3.627023, -10.739445)
  arc A41 (-3.627023, -10.739445) -> (-3.783579, -10.515859) centre (-3.880781, -10.750524) ccw
  line L25 (-3.783579, -10.515859) -> (-4.760441, -10.11123)
  arc A42 (-4.760441, -10.11123) -> (-5.029242, -10.158627) centre (-4.857642, -10.345895) ccw
  line L26 (-5.029242, -10.158627) -> (-5.808735, -10.872901)
  arc A43 (-6.104383, -10.907281) -> (-5.808735, -10.872901) centre (-5.980335, -10.685632) ccw
  arc A44 (-7.740967, -9.81375) -> (-6.104383, -10.907281) centre (0, 0) ccw
  arc A45 (-7.822344, -9.527451) -> (-7.740967, -9.81375) centre (-7.583662, -9.614324) ccw
  line L27 (-7.822344, -9.527451) -> (-7.46074, -8.533952)
  arc A46 (-7.46074, -8.533952) -> (-7.519817, -8.267474) centre (-7.699422, -8.447079) ccw
  line L28 (-7.519817, -8.267474) -> (-8.267474, -7.519817)
  arc A47 (-8.267474, -7.519817) -> (-8.533952, -7.46074) centre (-8.447079, -7.699422) ccw
  line L29 (-8.533952, -7.46074) -> (-9.527451, -7.822344)
  arc A48 (-9.81375, -7.740967) -> (-9.527451, -7.822344) centre (-9.614324, -7.583662) ccw
  arc A49 (-10.907281, -6.104383) -> (-9.81375, -7.740967) centre (0, 0) ccw
  arc A50 (-10.872901, -5.808735) -> (-10.907281, -6.104383) centre (-10.685632, -5.980335) ccw
  line L30 (-10.872901, -5.808735) -> (-10.158627, -5.029242)
  arc A51 (-10.158627, -5.029242) -> (-10.11123, -4.760441) centre (-10.345895, -4.857642) ccw
  line L31 (-10.11123, -4.760441) -> (-10.515859, -3.783579)
  arc A52 (-10.515859, -3.783579) -> (-10.739445, -3.627023) centre (-10.750524, -3.880781) ccw
  line L32 (-10.739445, -3.627023) -> (-11.795698, -3.580906)
  arc A53 (-12.029063, -3.396161) -> (-11.795698, -3.580906) centre (-11.784619, -3.327148) ccw
  arc A54 (-12.41306, -1.465679) -> (-12.029063, -3.396161) centre (0, 0) ccw
  arc A55 (-12.268157, -1.205693) -> (-12.41306, -1.465679) centre (-12.160812, -1.435895) ccw
  line L33 (-12.268157, -1.205693) -> (-11.309955, -0.758876)
  arc A56 (-11.309955, -0.758876) -> (-11.1633, -0.528673) centre (-11.4173, -0.528673) ccw
  line L34 (-11.1633, -0.528673) -> (-11.1633, 0.528673)
  arc A57 (-11.1633, 0.528673) -> (-11.309955, 0.758876) centre (-11.4173, 0.528673) ccw
  line L35 (-11.309955, 0.758876) -> (-12.268157, 1.205693)
  arc A58 (-12.41306, 1.465679) -> (-12.268157, 1.205693) centre (-12.160812, 1.435895) ccw
  arc A59 (-12.029063, 3.396161) -> (-12.41306, 1.465679) centre (0, 0) ccw
  arc A60 (-11.795698, 3.580906) -> (-12.029063, 3.396161) centre (-11.784619, 3.327148) ccw
  line L36 (-11.795698, 3.580906) -> (-10.739445, 3.627023)
  arc A61 (-10.739445, 3.627023) -> (-10.515859, 3.783579) centre (-10.750524, 3.880781) ccw
  line L37 (-10.515859, 3.783579) -> (-10.11123, 4.760441)
  arc A62 (-10.11123, 4.760441) -> (-10.158627, 5.029242) centre (-10.345895, 4.857642) ccw
  line L38 (-10.158627, 5.029242) -> (-10.872901, 5.808735)
  arc A63 (-10.907281, 6.104383) -> (-10.872901, 5.808735) centre (-10.685632, 5.980335) ccw
  arc A64 (-9.81375, 7.740967) -> (-10.907281, 6.104383) centre (0, 0) ccw
  arc A65 (-9.527451, 7.822344) -> (-9.81375, 7.740967) centre (-9.614324, 7.583662) ccw
  line L39 (-9.527451, 7.822344) -> (-8.533952, 7.46074)
  arc A66 (-8.533952, 7.46074) -> (-8.267474, 7.519817) centre (-8.447079, 7.699422) ccw
  line L40 (-8.267474, 7.519817) -> (-7.519817, 8.267474)
  arc A67 (-7.519817, 8.267474) -> (-7.46074, 8.533952) centre (-7.699422, 8.447079) ccw
  line L41 (-7.46074, 8.533952) -> (-7.822344, 9.527451)
  arc A68 (-7.740967, 9.81375) -> (-7.822344, 9.527451) centre (-7.583662, 9.614324) ccw
  arc A69 (-6.104383, 10.907281) -> (-7.740967, 9.81375) centre (0, 0) ccw
  arc A70 (-5.808735, 10.872901) -> (-6.104383, 10.907281) centre (-5.980335, 10.685632) ccw
  line L42 (-5.808735, 10.872901) -> (-5.029242, 10.158627)
  arc A71 (-5.029242, 10.158627) -> (-4.760441, 10.11123) centre (-4.857642, 10.345895) ccw
  line L43 (-4.760441, 10.11123) -> (-3.783579, 10.515859)
  arc A72 (-3.783579, 10.515859) -> (-3.627023, 10.739445) centre (-3.880781, 10.750524) ccw
  line L44 (-3.627023, 10.739445) -> (-3.580906, 11.795698)
  arc A73 (-3.396161, 12.029063) -> (-3.580906, 11.795698) centre (-3.327148, 11.784619) ccw
  arc A74 (-1.465679, 12.41306) -> (-3.396161, 12.029063) centre (0, 0) ccw
  arc A75 (-1.205693, 12.268157) -> (-1.465679, 12.41306) centre (-1.435895, 12.160812) ccw
  line L45 (-1.205693, 12.268157) -> (-0.758876, 11.309955)
  arc A76 (-0.758876, 11.309955) -> (-0.528673, 11.1633) centre (-0.528673, 11.4173) ccw
  line L46 (-0.528673, 11.1633) -> (0.528673, 11.1633)
  arc A77 (0.528673, 11.1633) -> (0.758876, 11.309955) centre (0.528673, 11.4173) ccw
  line L47 (0.758876, 11.309955) -> (1.205693, 12.268157)
  arc A78 (1.465679, 12.41306) -> (1.205693, 12.268157) centre (1.435895, 12.160812) ccw
  arc A79 (3.396161, 12.029063) -> (1.465679, 12.41306) centre (0, 0) ccw
  arc A80 (3.580906, 11.795698) -> (3.396161, 12.029063) centre (3.327148, 11.784619) ccw
  circle A81 centre (0, 0) radius 12.5
  dimension "d45" = 25
  dimension "d46" = 0
  dimension "d47" = 0
  dimension "d48" = 0
  dimension "d49" = 0
  constraints: 160 point on circle, 96 end point, 82 centre point, 2 coincident
  measures "d45" diameter of A81
  measures "d46" distance of point (0, 0) A4.centre
  measures "d47" distance of point (0, 0) A4.centre
  measures "d48" distance of point (0, 0) A0.centre
  measures "d49" distance of point (0, 0) A0.centre
extrude "Extrusion5" cut sketch "Sketch6" along normal blind 11.25 contours A80 A81 A3 L2 A2 L1 A1 L0 | A78 L47 A77 L46 A76 L45 A75 A81 | A81 A8 L5 A7 L4 A6 L3 A5 | A73 L44 A72 L43 A71 L42 A70 A81 | A81 A13 L8 A12 L7 A11 L6 A10 | A68 L41 A67 L40 A66 L39 A65 A81 | A81 A18 L11 A17 L10 A16 L9 A15 | A63 L38 A62 L37 A61 L36 A60 A81 | A58 L35 A57 L34 A56 L33 A55 A81 | A81 A23 L14 A22 L13 A21 L12 A20 | A53 L32 A52 L31 A51 L30 A50 A81 | A81 A28 L17 A27 L16 A26 L15 A25 | A48 L29 A47 L28 A46 L27 A45 A81 | A81 A33 L20 A32 L19 A31 L18 A30 | A43 L26 A42 L25 A41 L24 A40 A81 | A81 A38 L23 A37 L22 A36 L21 A35
body "Solid1"
